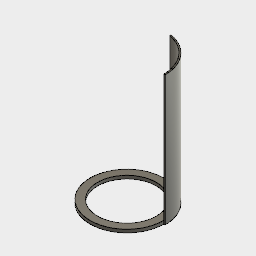
Gelatin_Mold_Remover v4 (Autodesk Fusion 360 design; units mm, degrees)
Autodesk Fusion 360 part; units mm, degrees
sketch "Sketch1" plane through (0, 0, 0) normal (0, 1, 0) x (1, 0, 0)
  circle A0 centre (0, 0) radius 34
  line L0 (0, 0) -> (35.25, 0)
  arc A1 (35.25, 0) -> (6.1211, 34.7145) centre (0, 0) ccw
  line L1 (0, 0) -> (6.1211, 34.7145)
  dimension "d1" = 68
  dimension "d15" = 70.5
  dimension "d19" = 80
  measures "d1" diameter of A0
  measures "d15" diameter of A1
  measures "d19" angle of L0 L1
extrude "Extrude1" add sketch "Sketch1" along normal blind 3 contours A0 L0 L1 | A0 L0 L1
extrude "Extrude2" add sketch "Sketch1" along normal blind 3 contours A0 L0 L1 picked at (22.5426, -1.6722)
sketch "Sketch2" plane through (0, 3, 0) normal (0, 1, 0) x (-1, 0, 0)
  circle A0 centre (0, 0) radius 34
  circle A1 centre (0, 0) radius 34
  circle A2 centre (0, 0) radius 27
  circle A3 centre (0, 0) radius 34
  dimension "d10" = 7
extrude "Extrude4" cut sketch "Sketch2" against normal blind 3 contours A2
extrude "Extrude5" add sketch "Sketch1" along normal blind 120 contours A0 L0 A1 L1
